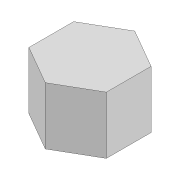
# Autodesk Inventor part: M3_lock_nut
Saved by Autodesk Inventor 2022 (Build 260153000, 153)
## iProperties
Created: 2022-07-02
Part Number: M3_lock_nut
Material: Generic
Document SubType Name: Modeling
Designer: dell
Density: 1 g/cm^3
Appearance: Default
Author: dell
Autodesk Inventor part; units mm, degrees
ref_plane "YZ Plane" through (0, 0, 0) normal (1, 0, 0) x (0, 1, 0)
ref_plane "XZ Plane" through (0, 0, 0) normal (0, 1, 0) x (-1, 0, 0)
ref_plane "XY Plane" through (0, 0, 0) normal (0, 0, 1) x (1, 0, 0)
sketch "Sketch1" plane through (0, 0, 0) normal (0, 1, 0) x (-1, 0, 0)
  line L0 (0, -3.1177) -> (-2.7, -1.5588)
  line L1 (-2.7, -1.5588) -> (-2.7, 1.5588)
  line L2 (-2.7, 1.5588) -> (0, 3.1177)
  line L3 (0, 3.1177) -> (2.7, 1.5588)
  line L4 (2.7, 1.5588) -> (2.7, -1.5588)
  line L5 (2.7, -1.5588) -> (0, -3.1177)
  point P0 (0, 0)
  point P1 (0, 0)
  dimension "d0" = 5.4
  constraints: 12 end point, 1 coincident, 13 other
  measures "d0" distance between parallel lines of L1 L4
extrude "Extrusion1" add sketch "Sketch1" along normal blind 4
body "Solid1"
